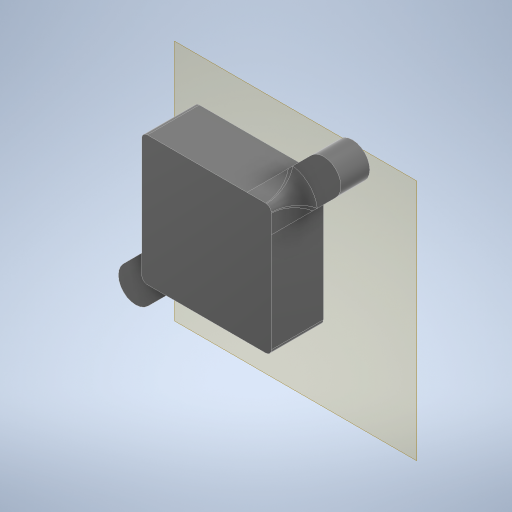
# Autodesk Inventor part: base
Saved by Autodesk Inventor 2023 (Build 270158000, 158)
## iProperties
Created: 2023-08-21
Part Number: base
Material: ABS Plastic
Document SubType Name: Modeling
Designer: chriboehm
Density: 1.06 g/cm^3
Appearance: Smooth - White
Author: chriboehm
Autodesk Inventor part; units mm, degrees
ref_plane "YZ Plane" through (0, 0, 0) normal (1, 0, 0) x (0, 1, 0)
ref_plane "XZ Plane" through (0, 0, 0) normal (0, 1, 0) x (-1, 0, 0)
ref_plane "XY Plane" through (0, 0, 0) normal (0, 0, 1) x (1, 0, 0)
ref_plane "Work Plane1" through (12.8382, -4.6513, 0) normal (0, 0, 1) x (1, 0, 0)
sketch "Sketch1" plane through (12.8382, -4.6513, 0) normal (0, 0, 1) x (1, 0, 0)
  circle A0 centre (-91.5002, -74.0108) radius 6
  circle A1 centre (-26.3324, -8.8429) radius 6
  ellipse E0 centre (-91.5002, -74.0108) end of major axis (-87.52, -70.0305) minor radius 5.6 (-97.1147, -74.0397) -> (-91.5291, -79.6253) ccw projected
  line L0 (-67.9442, -79.6253) -> (-91.5291, -79.6253) projected
  line L1 (-67.9442, -79.6253) -> (-49.8884, -79.6253) projected
  line L2 (-26.3034, -79.6253) -> (-49.8884, -79.6253) projected
  ellipse E1 centre (-26.3324, -74.0108) end of major axis (-22.3521, -77.991) minor radius 5.6 (-26.3034, -79.6253) -> (-20.7179, -74.0397) ccw projected
  line L3 (-20.7179, -8.814) -> (-20.7179, -74.0397) projected
  ellipse E2 centre (-26.3324, -8.8429) end of major axis (-22.3521, -4.8627) minor radius 5.6 (-20.7179, -8.814) -> (-26.3034, -3.2284) ccw projected
  line L4 (-91.5291, -3.2284) -> (-26.3034, -3.2284) projected
  ellipse E3 centre (-91.5002, -8.8429) end of major axis (-87.52, -12.8231) minor radius 5.6 (-91.5291, -3.2284) -> (-97.1147, -8.814) ccw projected
  line L5 (-97.1147, -74.0397) -> (-97.1147, -8.814) projected
  line L6 (-79.4163, -63.9268) -> (-38.4163, -63.9268)
  line L7 (-36.4163, -61.9268) -> (-36.4163, -20.9268)
  line L8 (-38.4163, -18.9268) -> (-79.4163, -18.9268)
  line L9 (-81.4163, -20.9268) -> (-81.4163, -61.9268)
  line L10 (-58.9163, -79.6253) -> (-58.9163, -3.2284)
  line L11 (-97.1147, -41.4268) -> (-20.7179, -41.4268)
  arc A2 (-81.4163, -61.9268) -> (-79.4163, -63.9268) centre (-79.4163, -61.9268) ccw
  arc A3 (-38.4163, -63.9268) -> (-36.4163, -61.9268) centre (-38.4163, -61.9268) ccw
  arc A4 (-36.4163, -20.9268) -> (-38.4163, -18.9268) centre (-38.4163, -20.9268) ccw
  arc A5 (-79.4163, -18.9268) -> (-81.4163, -20.9268) centre (-79.4163, -20.9268) ccw
  line L12 (-87.2576, -78.2534) -> (-22.0897, -13.0855)
  line L13 (-95.7429, -69.7681) -> (-30.575, -4.6003)
  point P0 (-12.8382, 4.6513)
  point P1 (-81.4163, -63.9268)
  point P2 (-36.4163, -18.9268)
  point P3 (-36.4163, -63.9268)
  point P4 (-72.931, -63.9268)
  point P5 (-36.4163, -27.4121)
  point P6 (-44.9016, -18.9268)
  point P7 (-81.4163, -55.4416)
  point P8 (-29.8782, -23.5781)
  point P9 (-75.1162, -63.9268)
  dimension "d0" = 12
  dimension "d1" = 12
  dimension "d2" = 45
  dimension "d3" = 45
  dimension "d4" = 2
  constraints: 16 end point, 12 point on circle, 12 tangent, 6 centre point, 6 point on line, 4 midpoint, 3 equal radius, 2 parallel, 1 horizontal, 1 perpendicular, 8 other
  measures "d0" diameter of A1
  measures "d1" diameter of A0
  measures "d2" distance of point (-81.416, -63.927) point (-36.416, -63.927)
  measures "d3" distance of point (-36.416, -63.927) point (-36.416, -18.927)
  measures "d4" radius of A2
extrude "Extrusion1" add sketch "Sketch1" along normal blind 18 contours A0 L0 E0 L5 | A0 L13 L9 A2 L6 L12 | L5 E0 L0 A0 | L13 L11 L10 L12 L6 A2 L9 | L9 L11 L13 | L12 L10 L6 | L9 A5 L8 L10 L13 L11 | L13 L10 L11 | L10 L12 L11 L7 A3 L6 | L10 L11 L12 | L10 L13 L8 A4 L7 L12 L11 | L10 L8 L13 | L12 L7 L11 | L13 A1 L12 L7 A4 L8 | A1 L4 E2 L3 | A1 L3 E2 L4
sketch "Sketch2" plane through (12.8382, -4.6513, 18) normal (0, 0, 1) x (1, 0, 0)
  line L0 (-44.9016, -18.9268) -> (-79.4163, -18.9268) projected
  arc A0 (-79.4163, -18.9268) -> (-81.4163, -20.9268) centre (-79.4163, -20.9268) ccw projected
  line L1 (-81.4163, -20.9268) -> (-81.4163, -55.4416) projected
  line L2 (-36.4163, -61.9268) -> (-36.4163, -27.4121) projected
  arc A1 (-38.4163, -63.9268) -> (-36.4163, -61.9268) centre (-38.4163, -61.9268) ccw projected
  line L3 (-72.931, -63.9268) -> (-38.4163, -63.9268) projected
  line L4 (-62.1589, -18.9268) -> (-55.6737, -63.9268)
  line L5 (-36.4163, -44.6695) -> (-81.4163, -38.1842)
  line L6 (-44.9016, -18.9268) -> (-79.4163, -18.9268)
  line L7 (-81.4163, -20.9268) -> (-81.4163, -55.4416)
  arc A2 (-79.4163, -18.9268) -> (-81.4163, -20.9268) centre (-79.4163, -20.9268) ccw
  line L8 (-81.4163, -27.4121) -> (-81.4163, -61.9268)
  arc A3 (-81.4163, -61.9268) -> (-79.4163, -63.9268) centre (-79.4163, -61.9268) ccw
  line L9 (-79.4163, -63.9268) -> (-44.9016, -63.9268)
  line L10 (-72.931, -63.9268) -> (-38.4163, -63.9268)
  arc A4 (-38.4163, -63.9268) -> (-36.4163, -61.9268) centre (-38.4163, -61.9268) ccw
  line L11 (-36.4163, -61.9268) -> (-36.4163, -27.4121)
  line L12 (-36.4163, -55.4416) -> (-36.4163, -20.9268)
  arc A5 (-36.4163, -20.9268) -> (-38.4163, -18.9268) centre (-38.4163, -20.9268) ccw
  line L13 (-38.4163, -18.9268) -> (-72.931, -18.9268)
  line L14 (-81.4163, -55.4416) -> (-100.4764, -69.4227)
  line L15 (-100.4764, -69.4227) -> (-100.4764, -80.6902)
  line L16 (-100.4764, -80.6902) -> (-89.2076, -83.945)
  line L17 (-89.2076, -83.945) -> (-75.1931, -71.7586)
  line L18 (-75.1931, -71.7586) -> (-72.931, -63.9268)
  line L19 (-44.9016, -18.9268) -> (-41.3617, -6.671)
  line L20 (-41.3617, -6.671) -> (-27.2892, 1.0126)
  line L21 (-27.2892, 1.0126) -> (-19.5179, 0.2355)
  line L22 (-19.5179, 0.2355) -> (-4.3296, -12.1655)
  line L23 (-4.3296, -12.1655) -> (-5.4222, -23.0912)
  line L24 (-5.4222, -23.0912) -> (-36.4163, -27.4121)
  point P0 (-12.8382, 4.6513)
  point P1 (-58.9163, -41.4268)
  point P2 (-81.4163, -55.4416)
  point P3 (-72.931, -63.9268)
  point P4 (-36.4163, -27.4121)
  point P5 (-43.7192, -14.8334)
  point P6 (-32.0634, -23.5781)
  point P7 (-25.5781, -68.5781)
  point P8 (-23.5781, -32.0634)
  point P9 (-32.0634, -23.5781)
  point P10 (-38.4163, -63.9268)
  dimension "d9" = 360
  constraints: 42 end point, 8 point on circle, 5 midpoint, 4 centre point, 3 perpendicular, 1 collinear, 1 tangent, 1 vertical, 33 other
extrude "Extrusion2" cut sketch "Sketch2" against normal blind 8 contours L19 L20 L21 L22 L23 L24 L12 A5 L13 | L18 L17 L16 L15 L14 L8 A3 L9
fillet "Fillet1" radius 8 6 edges at (-28.8207, -23.5781, 10) (-23.5781, -28.8207, 10) (-24.1639, -24.1639, 10) (-63.3355, -68.5781, 10) (-68.5781, -63.3355, 10) (-67.9923, -67.9923, 10)
equation "\"d1\" = d0"
equation "\"d3\" = d2"
body "Solid1"
